Autodesk Inventor part; units mm, degrees
(part 2 of 3)
  line L434 (6.5872, -21.6405) -> (5.7652, -19.2795)
  line L435 (1.8366, -22.5787) -> (2.09, -20.0135)
  line L436 (2.09, -20.0135) -> (2.4587, -19.9586)
  line L437 (2.4587, -19.9586) -> (3.2669, -21.9358)
  line L438 (3.2669, -21.9358) -> (3.4507, -19.8111)
  line L439 (3.4507, -19.8111) -> (3.8154, -19.7568)
  line L440 (3.8154, -19.7568) -> (4.8144, -22.1357)
  line L441 (4.8144, -22.1357) -> (4.4758, -22.1861)
  line L442 (4.4758, -22.1861) -> (3.6739, -20.21)
  line L443 (3.6739, -20.21) -> (3.4858, -22.3333)
  line L444 (3.4858, -22.3333) -> (3.1512, -22.3831)
  line L445 (3.1512, -22.3831) -> (2.3457, -20.383)
  line L446 (2.3457, -20.383) -> (2.1593, -22.5307)
  line L447 (2.1593, -22.5307) -> (1.8366, -22.5787)
  line L448 (1.4387, -20.0798) -> (0.6427, -22.5951)
  line L449 (0.6427, -22.5951) -> (0.2335, -22.6027)
  line L450 (0.2335, -22.6027) -> (-0.6558, -20.1189)
  line L451 (-0.6558, -20.1189) -> (-0.3054, -20.1124)
  line L452 (-0.3054, -20.1124) -> (-0.0655, -20.807)
  line L453 (-0.0655, -20.807) -> (0.8886, -20.7891)
  line L454 (0.8886, -20.7891) -> (1.1024, -20.0861)
  line L455 (1.1024, -20.0861) -> (1.4387, -20.0798)
  line L456 (0.031, -21.0888) -> (0.4398, -22.2585)
  line L457 (0.4398, -22.2585) -> (0.8027, -21.0744)
  line L458 (0.8027, -21.0744) -> (0.031, -21.0888)
  line L459 (-2.9434, -22.4342) -> (-1.873, -20.0164)
  line L460 (-1.873, -20.0164) -> (-1.5158, -20.0469)
  line L461 (-1.5158, -20.0469) -> (-0.8703, -22.611)
  line L462 (-0.8703, -22.611) -> (-1.2256, -22.5807)
  line L463 (-1.2256, -22.5807) -> (-1.7395, -20.4528)
  line L464 (-1.7395, -20.4528) -> (-2.6063, -22.4629)
  line L465 (-2.6063, -22.4629) -> (-2.9434, -22.4342)
  line L466 (-2.9935, -19.8918) -> (-3.4527, -22.3492)
  line L467 (-3.4527, -22.3492) -> (-4.9901, -22.0619)
  line L468 (-4.9901, -22.0619) -> (-4.9358, -21.7712)
  line L469 (-4.9358, -21.7712) -> (-3.725, -21.9974)
  line L470 (-3.725, -21.9974) -> (-3.5992, -21.3243)
  line L471 (-3.5992, -21.3243) -> (-4.7284, -21.1133)
  line L472 (-4.7284, -21.1133) -> (-4.674, -20.8226)
  line L473 (-4.674, -20.8226) -> (-3.5449, -21.0336)
  line L474 (-3.5449, -21.0336) -> (-3.3744, -20.1215)
  line L475 (-3.3744, -20.1215) -> (-4.5852, -19.8952)
  line L476 (-4.5852, -19.8952) -> (-4.5309, -19.6045)
  line L477 (-4.5309, -19.6045) -> (-2.9935, -19.8918)
  line L478 (-7.744, -18.5856) -> (-7.337, -18.7292)
  line L479 (-7.337, -18.7292) -> (-6.9228, -19.93)
  line L480 (-6.9228, -19.93) -> (-6.5636, -20.0567)
  line L481 (-6.5636, -20.0567) -> (-6.2327, -19.1186)
  line L482 (-6.2327, -19.1186) -> (-5.9194, -19.2291)
  line L483 (-5.9194, -19.2291) -> (-6.7509, -21.5868)
  line L484 (-6.7509, -21.5868) -> (-7.3585, -21.3725)
  spline S195 degree 2 poles (-7.3585, -21.3725) (-7.561, -21.3011) (-7.8187, -21.1608) (-7.9146, -21.0367) knots 0 0 0 1 2 2 2
  spline S196 degree 2 poles (-7.9146, -21.0367) (-8.0105, -20.9127) (-8.0655, -20.6119) (-8.0001, -20.4266) knots 0 0 0 1 2 2 2
  spline S197 degree 2 poles (-8.0001, -20.4266) (-7.9092, -20.1686) (-7.5222, -19.912) (-7.2671, -19.9074) knots 0 0 0 1 2 2 2
  line L485 (-7.2671, -19.9074) -> (-7.744, -18.5856)
  spline S198 degree 2 poles (-7.6647, -20.5169) (-7.7011, -20.6201) (-7.6844, -20.8043) (-7.6261, -20.8828) knots 0 0 0 1 2 2 2
  spline S199 degree 2 poles (-7.6261, -20.8828) (-7.5748, -20.9504) (-7.4099, -21.0493) (-7.28, -21.0952) knots 0 0 0 1 2 2 2
  line L486 (-7.28, -21.0952) -> (-6.9685, -21.205)
  line L487 (-6.9685, -21.205) -> (-6.6559, -20.3185)
  line L488 (-6.6559, -20.3185) -> (-6.931, -20.2214)
  spline S200 degree 2 poles (-6.931, -20.2214) (-7.0667, -20.1736) (-7.2994, -20.1452) (-7.4002, -20.1935) knots 0 0 0 1 2 2 2
  spline S201 degree 2 poles (-7.4002, -20.1935) (-7.4919, -20.2342) (-7.6215, -20.3947) (-7.6647, -20.5169) knots 0 0 0 1 2 2 2
  line L489 (-7.9195, -18.4912) -> (-8.9844, -20.753)
  line L490 (-8.9844, -20.753) -> (-10.3995, -20.0869)
  line L491 (-10.3995, -20.0869) -> (-10.2735, -19.8192)
  line L492 (-10.2735, -19.8192) -> (-9.159, -20.3439)
  line L493 (-9.159, -20.3439) -> (-8.8674, -19.7244)
  line L494 (-8.8674, -19.7244) -> (-9.9066, -19.2351)
  line L495 (-9.9066, -19.2351) -> (-9.7807, -18.9675)
  line L496 (-9.7807, -18.9675) -> (-8.7414, -19.4568)
  line L497 (-8.7414, -19.4568) -> (-8.3461, -18.6173)
  line L498 (-8.3461, -18.6173) -> (-9.4606, -18.0926)
  line L499 (-9.4606, -18.0926) -> (-9.3346, -17.825)
  line L500 (-9.3346, -17.825) -> (-7.9195, -18.4912)
  spline S202 degree 2 poles (-11.9895, -17.6987) (-11.8118, -17.4061) (-11.2884, -17.0792) (-11.0094, -17.0685) knots 0 0 0 1 2 2 2
  spline S203 degree 2 poles (-11.0094, -17.0685) (-10.7846, -17.0653) (-10.4083, -17.199) (-10.1486, -17.3568) knots 0 0 0 1 2 2 2
  line L501 (-10.1486, -17.3568) -> (-9.6568, -17.6555)
  line L502 (-9.6568, -17.6555) -> (-10.9548, -19.7922)
  line L503 (-10.9548, -19.7922) -> (-11.4413, -19.4966)
  spline S204 degree 2 poles (-11.4413, -19.4966) (-11.7426, -19.3136) (-12.0307, -19.0153) (-12.1036, -18.862) knots 0 0 0 1 2 2 2
  spline S205 degree 2 poles (-12.1036, -18.862) (-12.2265, -18.6001) (-12.1788, -18.0104) (-11.9895, -17.6987) knots 0 0 0 1 2 2 2
  spline S206 degree 2 poles (-11.6955, -17.882) (-11.8449, -18.1279) (-11.8935, -18.5748) (-11.7924, -18.7713) knots 0 0 0 1 2 2 2
  spline S207 degree 2 poles (-11.7924, -18.7713) (-11.7192, -18.9082) (-11.498, -19.1256) (-11.3058, -19.2423) knots 0 0 0 1 2 2 2
  line L504 (-11.3058, -19.2423) -> (-11.0894, -19.3738)
  line L505 (-11.0894, -19.3738) -> (-10.0902, -17.7289)
  line L506 (-10.0902, -17.7289) -> (-10.3066, -17.5974)
  spline S208 degree 2 poles (-10.3066, -17.5974) (-10.4953, -17.4827) (-10.8178, -17.3698) (-10.9833, -17.3807) knots 0 0 0 1 2 2 2
  spline S209 degree 2 poles (-10.9833, -17.3807) (-11.1932, -17.3907) (-11.5441, -17.6327) (-11.6955, -17.882) knots 0 0 0 1 2 2 2
  spline S210 degree 2 poles (-12.2898, -15.8424) (-12.1153, -15.9778) (-11.9268, -16.2702) (-11.9064, -16.4322) knots 0 0 0 1 2 2 2
  spline S211 degree 2 poles (-11.9064, -16.4322) (-11.8818, -16.6154) (-12.0205, -16.9693) (-12.1844, -17.1806) knots 0 0 0 1 2 2 2
  line L507 (-12.1844, -17.1806) -> (-13.1407, -18.4132)
  line L508 (-13.1407, -18.4132) -> (-13.4032, -18.2095)
  line L509 (-13.4032, -18.2095) -> (-12.4469, -16.977)
  spline S212 degree 2 poles (-12.4469, -16.977) (-12.3401, -16.8393) (-12.2313, -16.6263) (-12.2225, -16.5126) knots 0 0 0 1 2 2 2
  spline S213 degree 2 poles (-12.2225, -16.5126) (-12.2133, -16.3916) (-12.3324, -16.1684) (-12.4637, -16.0665) knots 0 0 0 1 2 2 2
  spline S214 degree 2 poles (-12.4637, -16.0665) (-12.5869, -15.9709) (-12.8423, -15.9035) (-12.9573, -15.9426) knots 0 0 0 1 2 2 2
  spline S215 degree 2 poles (-12.9573, -15.9426) (-13.0652, -15.9793) (-13.2433, -16.1361) (-13.3464, -16.2689) knots 0 0 0 1 2 2 2
  line L510 (-13.3464, -16.2689) -> (-14.3076, -17.5078)
  line L511 (-14.3076, -17.5078) -> (-14.5701, -17.3042)
  line L512 (-14.5701, -17.3042) -> (-13.6138, -16.0717)
  spline S216 degree 2 poles (-13.6138, -16.0717) (-13.4536, -15.8652) (-13.1419, -15.6352) (-12.958, -15.6163) knots 0 0 0 1 2 2 2
  spline S217 degree 2 poles (-12.958, -15.6163) (-12.7915, -15.5968) (-12.4723, -15.7009) (-12.2898, -15.8424) knots 0 0 0 1 2 2 2
  spline S218 degree 2 poles (-14.0647, -14.3028) (-13.8897, -14.4716) (-13.7075, -14.8752) (-13.7135, -15.0974) knots 0 0 0 1 2 2 2
  spline S219 degree 2 poles (-13.7135, -15.0974) (-13.718, -15.3181) (-13.9374, -15.782) (-14.1568, -16.0095) knots 0 0 0 1 2 2 2
  spline S220 degree 2 poles (-14.1568, -16.0095) (-14.3747, -16.2356) (-14.8133, -16.46) (-15.0423, -16.4785) knots 0 0 0 1 2 2 2
  spline S221 degree 2 poles (-15.0423, -16.4785) (-15.2669, -16.4955) (-15.6838, -16.3383) (-15.8661, -16.1625) knots 0 0 0 1 2 2 2
  spline S222 degree 2 poles (-15.8661, -16.1625) (-15.9566, -16.0753) (-16.0902, -15.8958) (-16.1376, -15.8107) knots 0 0 0 1 2 2 2
  spline S223 degree 2 poles (-16.1376, -15.8107) (-16.1777, -15.7355) (-16.2467, -15.5648) (-16.2756, -15.4751) knots 0 0 0 1 2 2 2
  line L513 (-16.2756, -15.4751) -> (-15.9971, -15.1863)
  line L514 (-15.9971, -15.1863) -> (-15.9782, -15.2046)
  spline S224 degree 2 poles (-15.9782, -15.2046) (-15.9742, -15.2647) (-15.9538, -15.442) (-15.9203, -15.5503) knots 0 0 0 1 2 2 2
  spline S225 degree 2 poles (-15.9203, -15.5503) (-15.8883, -15.6543) (-15.7728, -15.8585) (-15.6678, -15.9597) knots 0 0 0 1 2 2 2
  spline S226 degree 2 poles (-15.6678, -15.9597) (-15.5526, -16.0708) (-15.2556, -16.1743) (-15.0911, -16.1584) knots 0 0 0 1 2 2 2
  spline S227 degree 2 poles (-15.0911, -16.1584) (-14.9267, -16.1396) (-14.5735, -15.9426) (-14.4061, -15.7691) knots 0 0 0 1 2 2 2
  spline S228 degree 2 poles (-14.4061, -15.7691) (-14.2276, -15.5839) (-14.0592, -15.2312) (-14.0479, -15.0648) knots 0 0 0 1 2 2 2
  spline S229 degree 2 poles (-14.0479, -15.0648) (-14.038, -14.9027) (-14.1535, -14.6168) (-14.2673, -14.5071) knots 0 0 0 1 2 2 2
  spline S230 degree 2 poles (-14.2673, -14.5071) (-14.3708, -14.4073) (-14.5965, -14.2882) (-14.7016, -14.26) knots 0 0 0 1 2 2 2
  spline S231 degree 2 poles (-14.7016, -14.26) (-14.8038, -14.2347) (-14.9775, -14.2192) (-15.0319, -14.2202) knots 0 0 0 1 2 2 2
  line L515 (-15.0319, -14.2202) -> (-15.0494, -14.2033)
  line L516 (-15.0494, -14.2033) -> (-14.7738, -13.9175)
  spline S232 degree 2 poles (-14.7738, -13.9175) (-14.6873, -13.9474) (-14.533, -13.9976) (-14.4362, -14.046) knots 0 0 0 1 2 2 2
  spline S233 degree 2 poles (-14.4362, -14.046) (-14.3321, -14.0957) (-14.1726, -14.1988) (-14.0647, -14.3028) knots 0 0 0 1 2 2 2
  line L517 (-14.858, -13.5603) -> (-16.763, -15.1793)
  line L518 (-16.763, -15.1793) -> (-17.7758, -13.9875)
  line L519 (-17.7758, -13.9875) -> (-17.5505, -13.7959)
  line L520 (-17.5505, -13.7959) -> (-16.7528, -14.7345)
  line L521 (-16.7528, -14.7345) -> (-16.231, -14.2911)
  line L522 (-16.231, -14.2911) -> (-16.9749, -13.4158)
  line L523 (-16.9749, -13.4158) -> (-16.7495, -13.2243)
  line L524 (-16.7495, -13.2243) -> (-16.0056, -14.0996)
  line L525 (-16.0056, -14.0996) -> (-15.2986, -13.4987)
  line L526 (-15.2986, -13.4987) -> (-16.0962, -12.5601)
  line L527 (-16.0962, -12.5601) -> (-15.8709, -12.3685)
  line L528 (-15.8709, -12.3685) -> (-14.858, -13.5603)
  line L529 (-17.1888, -10.4852) -> (-16.9439, -10.8405)
  line L530 (-16.9439, -10.8405) -> (-17.3146, -12.0556)
  line L531 (-17.3146, -12.0556) -> (-17.0984, -12.3692)
  line L532 (-17.0984, -12.3692) -> (-16.2794, -11.8047)
  line L533 (-16.2794, -11.8047) -> (-16.0908, -12.0783)
  line L534 (-16.0908, -12.0783) -> (-18.1493, -13.497)
  line L535 (-18.1493, -13.497) -> (-18.5149, -12.9666)
  spline S234 degree 2 poles (-18.5149, -12.9666) (-18.6367, -12.7897) (-18.7628, -12.5248) (-18.7674, -12.368) knots 0 0 0 1 2 2 2
  spline S235 degree 2 poles (-18.7674, -12.368) (-18.7721, -12.2113) (-18.6398, -11.9356) (-18.478, -11.8241) knots 0 0 0 1 2 2 2
  spline S236 degree 2 poles (-18.478, -11.8241) (-18.2528, -11.6689) (-17.7889, -11.6887) (-17.5798, -11.8349) knots 0 0 0 1 2 2 2
  line L536 (-17.5798, -11.8349) -> (-17.1888, -10.4852)
  spline S237 degree 2 poles (-18.2597, -12.0944) (-18.3498, -12.1565) (-18.4446, -12.3153) (-18.4436, -12.4131) knots 0 0 0 1 2 2 2
  spline S238 degree 2 poles (-18.4436, -12.4131) (-18.4417, -12.4979) (-18.3665, -12.6749) (-18.2883, -12.7883) knots 0 0 0 1 2 2 2
  line L537 (-18.2883, -12.7883) -> (-18.1009, -13.0602)
  line L538 (-18.1009, -13.0602) -> (-17.3269, -12.5267)
  line L539 (-17.3269, -12.5267) -> (-17.4925, -12.2865)
  spline S239 degree 2 poles (-17.4925, -12.2865) (-17.5741, -12.1681) (-17.7457, -12.0083) (-17.8556, -11.9881) knots 0 0 0 1 2 2 2
  spline S240 degree 2 poles (-17.8556, -11.9881) (-17.9537, -11.9671) (-18.153, -12.0208) (-18.2597, -12.0944) knots 0 0 0 1 2 2 2
  line L540 (-20.4598, -8.1233) -> (-18.5574, -7.7669)
  line L541 (-18.5574, -7.7669) -> (-18.4348, -8.0316)
  line L542 (-18.4348, -8.0316) -> (-19.5549, -9.055)
  line L543 (-19.5549, -9.055) -> (-18.0508, -8.8607)
  line L544 (-18.0508, -8.8607) -> (-17.9291, -9.1236)
  line L545 (-17.9291, -9.1236) -> (-19.4296, -10.3477)
  line L546 (-19.4296, -10.3477) -> (-19.5675, -10.0499)
  line L547 (-19.5675, -10.0499) -> (-18.389, -9.1379)
  line L548 (-18.389, -9.1379) -> (-19.8936, -9.3458)
  line L549 (-19.8936, -9.3458) -> (-20.0034, -9.1086)
  line L550 (-20.0034, -9.1086) -> (-18.8769, -8.0846)
  line L551 (-18.8769, -8.0846) -> (-20.3261, -8.4119)
  line L552 (-20.3261, -8.4119) -> (-20.4598, -8.1233)
  line L553 (-18.9331, -6.76) -> (-18.8245, -7.0568)
  line L554 (-18.8245, -7.0568) -> (-20.5863, -7.7015)
  line L555 (-20.5863, -7.7015) -> (-20.6949, -7.4047)
  line L556 (-20.6949, -7.4047) -> (-18.9331, -6.76)
  line L557 (-20.9956, -7.491) -> (-20.8723, -7.8278)
  line L558 (-20.8723, -7.8278) -> (-21.1805, -7.9406)
  line L559 (-21.1805, -7.9406) -> (-21.3038, -7.6038)
  line L560 (-21.3038, -7.6038) -> (-20.9956, -7.491)
  spline S241 degree 2 poles (-19.2205, -5.7699) (-19.1439, -6.0155) (-19.3379, -6.3796) (-19.6415, -6.4744) knots 0 0 0 1 2 2 2
  line L561 (-19.6415, -6.4744) -> (-20.6336, -6.7842)
  line L562 (-20.6336, -6.7842) -> (-20.5702, -6.9872)
  line L563 (-20.5702, -6.9872) -> (-20.8197, -7.0651)
  line L564 (-20.8197, -7.0651) -> (-20.8831, -6.862)
  line L565 (-20.8831, -6.862) -> (-21.3975, -7.0227)
  line L566 (-21.3975, -7.0227) -> (-21.4917, -6.721)
  line L567 (-21.4917, -6.721) -> (-20.9773, -6.5604)
  line L568 (-20.9773, -6.5604) -> (-21.1506, -6.0053)
  line L569 (-21.1506, -6.0053) -> (-20.9011, -5.9275)
  line L570 (-20.9011, -5.9275) -> (-20.7278, -6.4825)
  line L571 (-20.7278, -6.4825) -> (-19.875, -6.2162)
  spline S242 degree 2 poles (-19.875, -6.2162) (-19.7396, -6.1739) (-19.5937, -6.1178) (-19.5402, -6.065) knots 0 0 0 1 2 2 2
  spline S243 degree 2 poles (-19.5402, -6.065) (-19.4925, -6.0204) (-19.4745, -5.881) (-19.5071, -5.7766) knots 0 0 0 1 2 2 2
  spline S244 degree 2 poles (-19.5071, -5.7766) (-19.53, -5.7031) (-19.6174, -5.5797) (-19.6406, -5.553) knots 0 0 0 1 2 2 2
  line L572 (-19.6406, -5.553) -> (-19.646, -5.5356)
  line L573 (-19.646, -5.5356) -> (-19.3753, -5.451)
  spline S245 degree 2 poles (-19.3753, -5.451) (-19.3255, -5.5289) (-19.2441, -5.6945) (-19.2205, -5.7699) knots 0 0 0 1 2 2 2
  line L574 (-19.7571, -3.7879) -> (-19.6861, -4.0959)
  line L575 (-19.6861, -4.0959) -> (-20.7285, -4.336)
  spline S246 degree 2 poles (-20.7285, -4.336) (-20.8549, -4.3651) (-21.0666, -4.4389) (-21.1235, -4.4894) knots 0 0 0 1 2 2 2
  spline S247 degree 2 poles (-21.1235, -4.4894) (-21.184, -4.5428) (-21.2202, -4.6925) (-21.1938, -4.807) knots 0 0 0 1 2 2 2
  spline S248 degree 2 poles (-21.1938, -4.807) (-21.1674, -4.9215) (-20.9891, -5.1362) (-20.8636, -5.2299) knots 0 0 0 1 2 2 2
  line L576 (-20.8636, -5.2299) -> (-19.4974, -4.9152)
  line L577 (-19.4974, -4.9152) -> (-19.4265, -5.2232)
  line L578 (-19.4265, -5.2232) -> (-21.9712, -5.8094)
  line L579 (-21.9712, -5.8094) -> (-22.0422, -5.5014)
  line L580 (-22.0422, -5.5014) -> (-21.1222, -5.2895)
  spline S249 degree 2 poles (-21.1222, -5.2895) (-21.2784, -5.1799) (-21.4701, -4.9434) (-21.5047, -4.7934) knots 0 0 0 1 2 2 2
  spline S250 degree 2 poles (-21.5047, -4.7934) (-21.5665, -4.5249) (-21.2812, -4.139) (-20.9436, -4.0612) knots 0 0 0 1 2 2 2
  line L581 (-20.9436, -4.0612) -> (-19.7571, -3.7879)
  spline S251 degree 2 poles (-20.0182, -1.2873) (-20.0002, -1.5297) (-20.1335, -1.952) (-20.286, -2.1137) knots 0 0 0 1 2 2 2
  spline S252 degree 2 poles (-20.286, -2.1137) (-20.4365, -2.2752) (-20.9093, -2.4748) (-21.2245, -2.4982) knots 0 0 0 1 2 2 2
  spline S253 degree 2 poles (-21.2245, -2.4982) (-21.5376, -2.5214) (-22.0142, -2.3963) (-22.1971, -2.2575) knots 0 0 0 1 2 2 2
  spline S254 degree 2 poles (-22.1971, -2.2575) (-22.3759, -2.1204) (-22.582, -1.7254) (-22.6007, -1.4728) knots 0 0 0 1 2 2 2
  spline S255 degree 2 poles (-22.6007, -1.4728) (-22.61, -1.3475) (-22.59, -1.1246) (-22.5686, -1.0296) knots 0 0 0 1 2 2 2
  spline S256 degree 2 poles (-22.5686, -1.0296) (-22.5483, -0.9468) (-22.486, -0.7736) (-22.4477, -0.6875) knots 0 0 0 1 2 2 2
  line L582 (-22.4477, -0.6875) -> (-22.0477, -0.6578)
  line L583 (-22.0477, -0.6578) -> (-22.0457, -0.684)
  spline S257 degree 2 poles (-22.0457, -0.684) (-22.0828, -0.7315) (-22.1858, -0.8773) (-22.233, -0.9803) knots 0 0 0 1 2 2 2
  spline S258 degree 2 poles (-22.233, -0.9803) (-22.2785, -1.0792) (-22.3285, -1.3084) (-22.3177, -1.4538) knots 0 0 0 1 2 2 2
  spline S259 degree 2 poles (-22.3177, -1.4538) (-22.3059, -1.6135) (-22.1534, -1.8886) (-22.0202, -1.9864) knots 0 0 0 1 2 2 2
  spline S260 degree 2 poles (-22.0202, -1.9864) (-21.8851, -2.082) (-21.4905, -2.1705) (-21.2501, -2.1527) knots 0 0 0 1 2 2 2
  spline S261 degree 2 poles (-21.2501, -2.1527) (-20.9935, -2.1337) (-20.6329, -1.983) (-20.5136, -1.8665) knots 0 0 0 1 2 2 2
  spline S262 degree 2 poles (-20.5136, -1.8665) (-20.3981, -1.7522) (-20.2937, -1.4621) (-20.3054, -1.3045) knots 0 0 0 1 2 2 2
  spline S263 degree 2 poles (-20.3054, -1.3045) (-20.3161, -1.1611) (-20.4049, -0.9219) (-20.4645, -0.8308) knots 0 0 0 1 2 2 2
  spline S264 degree 2 poles (-20.4645, -0.8308) (-20.5238, -0.7438) (-20.6429, -0.6165) (-20.6841, -0.581) knots 0 0 0 1 2 2 2
  line L584 (-20.6841, -0.581) -> (-20.6859, -0.5567)
  line L585 (-20.6859, -0.5567) -> (-20.2899, -0.5273)
  spline S265 degree 2 poles (-20.2899, -0.5273) (-20.2454, -0.6073) (-20.1639, -0.7476) (-20.1239, -0.8482) knots 0 0 0 1 2 2 2
  spline S266 degree 2 poles (-20.1239, -0.8482) (-20.0795, -0.9546) (-20.0293, -1.1378) (-20.0182, -1.2873) knots 0 0 0 1 2 2 2
  line L586 (-20.0601, 1.7288) -> (-20.0731, 1.2975)
  line L587 (-20.0731, 1.2975) -> (-21.0913, 0.5378)
  line L588 (-21.0913, 0.5378) -> (-21.1028, 0.1571)
  line L589 (-21.1028, 0.1571) -> (-20.1085, 0.127)
  line L590 (-20.1085, 0.127) -> (-20.1186, -0.2051)
  line L591 (-20.1186, -0.2051) -> (-22.6174, -0.1295)
  line L592 (-22.6174, -0.1295) -> (-22.5979, 0.5145)
  spline S267 degree 2 poles (-22.5979, 0.5145) (-22.5914, 0.7291) (-22.5361, 1.0173) (-22.4471, 1.1463) knots 0 0 0 1 2 2 2
  spline S268 degree 2 poles (-22.4471, 1.1463) (-22.358, 1.2754) (-22.0882, 1.4192) (-21.8918, 1.4133) knots 0 0 0 1 2 2 2
  spline S269 degree 2 poles (-21.8918, 1.4133) (-21.6184, 1.405) (-21.2563, 1.1143) (-21.1744, 0.8727) knots 0 0 0 1 2 2 2
  line L593 (-21.1744, 0.8727) -> (-20.0601, 1.7288)
  spline S270 degree 2 poles (-21.8759, 1.0662) (-21.9853, 1.0695) (-22.1557, 0.9977) (-22.2128, 0.9183) knots 0 0 0 1 2 2 2
  spline S271 degree 2 poles (-22.2128, 0.9183) (-22.2615, 0.8488) (-22.3057, 0.6617) (-22.3098, 0.524) knots 0 0 0 1 2 2 2
  line L594 (-22.3098, 0.524) -> (-22.3198, 0.1939)
  line L595 (-22.3198, 0.1939) -> (-21.3802, 0.1655)
  line L596 (-21.3802, 0.1655) -> (-21.3714, 0.4571)
  spline S272 degree 2 poles (-21.3714, 0.4571) (-21.3671, 0.6009) (-21.4108, 0.8312) (-21.4873, 0.9126) knots 0 0 0 1 2 2 2
  spline S273 degree 2 poles (-21.4873, 0.9126) (-21.554, 0.9876) (-21.7463, 1.0623) (-21.8759, 1.0662) knots 0 0 0 1 2 2 2
  spline S274 degree 2 poles (-21.9722, 3.993) (-21.7874, 4.1095) (-21.2836, 4.1963) (-20.9748, 4.1516) knots 0 0 0 1 2 2 2
  spline S275 degree 2 poles (-20.9748, 4.1516) (-20.6741, 4.1081) (-20.2089, 3.8852) (-20.0654, 3.717) knots 0 0 0 1 2 2 2
  spline S276 degree 2 poles (-20.0654, 3.717) (-19.915, 3.5397) (-19.8089, 3.1129) (-19.844, 2.8703) knots 0 0 0 1 2 2 2
  spline S277 degree 2 poles (-19.844, 2.8703) (-19.8802, 2.6197) (-20.1087, 2.2433) (-20.2963, 2.121) knots 0 0 0 1 2 2 2
  spline S278 degree 2 poles (-20.2963, 2.121) (-20.4813, 2.0025) (-20.9866, 1.92) (-21.2913, 1.9641) knots 0 0 0 1 2 2 2
  spline S279 degree 2 poles (-21.2913, 1.9641) (-21.6021, 2.0091) (-22.053, 2.2319) (-22.2028, 2.3989) knots 0 0 0 1 2 2 2
  spline S280 degree 2 poles (-22.2028, 2.3989) (-22.3463, 2.5671) (-22.4585, 2.9948) (-22.4225, 3.2434) knots 0 0 0 1 2 2 2
  spline S281 degree 2 poles (-22.4225, 3.2434) (-22.3859, 3.496) (-22.1509, 3.8755) (-21.9722, 3.993) knots 0 0 0 1 2 2 2
  spline S282 degree 2 poles (-21.0244, 3.8087) (-21.2691, 3.8441) (-21.6634, 3.7927) (-21.8016, 3.7144) knots 0 0 0 1 2 2 2
  spline S283 degree 2 poles (-21.8016, 3.7144) (-21.9442, 3.6348) (-22.1125, 3.3766) (-22.1375, 3.2042) knots 0 0 0 1 2 2 2
  spline S284 degree 2 poles (-22.1375, 3.2042) (-22.1633, 3.0258) (-22.0779, 2.7391) (-21.9603, 2.6177) knots 0 0 0 1 2 2 2
  spline S285 degree 2 poles (-21.9603, 2.6177) (-21.8482, 2.5012) (-21.4823, 2.3418) (-21.2417, 2.307) knots 0 0 0 1 2 2 2
  spline S286 degree 2 poles (-21.2417, 2.307) (-20.7545, 2.2365) (-20.178, 2.5706) (-20.1284, 2.9135) knots 0 0 0 1 2 2 2
  spline S287 degree 2 poles (-20.1284, 2.9135) (-20.0788, 3.2564) (-20.5372, 3.7382) (-21.0244, 3.8087) knots 0 0 0 1 2 2 2
  spline S288 degree 2 poles (-19.4282, 4.9892) (-19.4958, 4.7262) (-19.7006, 4.3856) (-19.8209, 4.243) knots 0 0 0 1 2 2 2
  line L597 (-19.8209, 4.243) -> (-20.2251, 4.3469)
  line L598 (-20.2251, 4.3469) -> (-20.2191, 4.3704)
  spline S289 degree 2 poles (-20.2191, 4.3704) (-20.0291, 4.491) (-19.7608, 4.8509) (-19.7129, 5.0373) knots 0 0 0 1 2 2 2
  spline S290 degree 2 poles (-19.7129, 5.0373) (-19.6443, 5.3041) (-19.7958, 5.6339) (-19.9783, 5.6808) knots 0 0 0 1 2 2 2
  spline S291 degree 2 poles (-19.9783, 5.6808) (-20.1235, 5.7181) (-20.3409, 5.6213) (-20.4258, 5.4779) knots 0 0 0 1 2 2 2
  spline S292 degree 2 poles (-20.4258, 5.4779) (-20.486, 5.3742) (-20.5771, 5.1989) (-20.6482, 5.0686) knots 0 0 0 1 2 2 2
  spline S293 degree 2 poles (-20.6482, 5.0686) (-20.7139, 4.9516) (-20.8649, 4.7792) (-20.9651, 4.7234) knots 0 0 0 1 2 2 2
  spline S294 degree 2 poles (-20.9651, 4.7234) (-21.0647, 4.6695) (-21.3017, 4.6426) (-21.443, 4.6789) knots 0 0 0 1 2 2 2
  spline S295 degree 2 poles (-21.443, 4.6789) (-21.7373, 4.7546) (-22.0175, 5.3162) (-21.9262, 5.6713) knots 0 0 0 1 2 2 2
  spline S296 degree 2 poles (-21.9262, 5.6713) (-21.8737, 5.8754) (-21.7004, 6.2157) (-21.584, 6.351) knots 0 0 0 1 2 2 2
  line L599 (-21.584, 6.351) -> (-21.1995, 6.2521)
  line L600 (-21.1995, 6.2521) -> (-21.2055, 6.2286)
  spline S297 degree 2 poles (-21.2055, 6.2286) (-21.3412, 6.1401) (-21.591, 5.8194) (-21.642, 5.6212) knots 0 0 0 1 2 2 2
  spline S298 degree 2 poles (-21.642, 5.6212) (-21.6995, 5.3976) (-21.5607, 5.0669) (-21.39, 5.023) knots 0 0 0 1 2 2 2
  spline S299 degree 2 poles (-21.39, 5.023) (-21.237, 4.9837) (-21.0126, 5.0996) (-20.9321, 5.242) knots 0 0 0 1 2 2 2
  spline S300 degree 2 poles (-20.9321, 5.242) (-20.8784, 5.337) (-20.7315, 5.6151) (-20.6769, 5.7056) knots 0 0 0 1 2 2 2
  spline S301 degree 2 poles (-20.6769, 5.7056) (-20.5363, 5.9351) (-20.1687, 6.0875) (-19.943, 6.0294) knots 0 0 0 1 2 2 2
  spline S302 degree 2 poles (-19.943, 6.0294) (-19.7998, 5.9926) (-19.5549, 5.8062) (-19.4855, 5.6775) knots 0 0 0 1 2 2 2
  spline S303 degree 2 poles (-19.4855, 5.6775) (-19.4093, 5.5345) (-19.3712, 5.2109) (-19.4282, 4.9892) knots 0 0 0 1 2 2 2
  spline S304 degree 2 poles (-18.8663, 6.8126) (-18.9585, 6.5573) (-19.1947, 6.2377) (-19.3281, 6.1071) knots 0 0 0 1 2 2 2
  line L601 (-19.3281, 6.1071) -> (-19.7206, 6.249)
  line L602 (-19.7206, 6.249) -> (-19.7123, 6.2719)
  spline S305 degree 2 poles (-19.7123, 6.2719) (-19.5117, 6.3738) (-19.2105, 6.7066) (-19.1451, 6.8876) knots 0 0 0 1 2 2 2
  spline S306 degree 2 poles (-19.1451, 6.8876) (-19.0514, 7.1467) (-19.171, 7.4893) (-19.3481, 7.5534) knots 0 0 0 1 2 2 2
  spline S307 degree 2 poles (-19.3481, 7.5534) (-19.4891, 7.6044) (-19.7147, 7.5286) (-19.8129, 7.394) knots 0 0 0 1 2 2 2
  spline S308 degree 2 poles (-19.8129, 7.394) (-19.8827, 7.2964) (-19.99, 7.1305) (-20.0732, 7.0077) knots 0 0 0 1 2 2 2
  spline S309 degree 2 poles (-20.0732, 7.0077) (-20.1497, 6.8974) (-20.3164, 6.7401) (-20.4214, 6.6941) knots 0 0 0 1 2 2 2
  spline S310 degree 2 poles (-20.4214, 6.6941) (-20.5257, 6.6499) (-20.7642, 6.6456) (-20.9014, 6.6952) knots 0 0 0 1 2 2 2
  spline S311 degree 2 poles (-20.9014, 6.6952) (-21.1872, 6.7986) (-21.4128, 7.3842) (-21.2881, 7.7291) knots 0 0 0 1 2 2 2
  spline S312 degree 2 poles (-21.2881, 7.7291) (-21.2165, 7.9272) (-21.0116, 8.2495) (-20.8829, 8.3732) knots 0 0 0 1 2 2 2
  line L603 (-20.8829, 8.3732) -> (-20.5095, 8.2382)
  line L604 (-20.5095, 8.2382) -> (-20.5177, 8.2153)
  spline S313 degree 2 poles (-20.5177, 8.2153) (-20.6613, 8.1401) (-20.9404, 7.8446) (-21.01, 7.6522) knots 0 0 0 1 2 2 2
  spline S314 degree 2 poles (-21.01, 7.6522) (-21.0885, 7.435) (-20.9817, 7.0927) (-20.816, 7.0327) knots 0 0 0 1 2 2 2
  spline S315 degree 2 poles (-20.816, 7.0327) (-20.6674, 6.979) (-20.433, 7.0731) (-20.3393, 7.2073) knots 0 0 0 1 2 2 2
  spline S316 degree 2 poles (-20.3393, 7.2073) (-20.2768, 7.2967) (-20.1042, 7.5596) (-20.0412, 7.6445) knots 0 0 0 1 2 2 2
  spline S317 degree 2 poles (-20.0412, 7.6445) (-19.8794, 7.8596) (-19.499, 7.9763) (-19.2799, 7.8971) knots 0 0 0 1 2 2 2
  spline S318 degree 2 poles (-19.2799, 7.8971) (-19.1408, 7.8468) (-18.9147, 7.638) (-18.8579, 7.5033) knots 0 0 0 1 2 2 2
  spline S319 degree 2 poles (-18.8579, 7.5033) (-18.7956, 7.3537) (-18.7884, 7.0279) (-18.8663, 6.8126) knots 0 0 0 1 2 2 2
  line L605 (-17.0953, 10.637) -> (-17.3025, 10.2585)
  line L606 (-17.3025, 10.2585) -> (-18.5545, 10.0431)
  line L607 (-18.5545, 10.0431) -> (-18.7374, 9.709)
  line L608 (-18.7374, 9.709) -> (-17.8648, 9.2313)
  line L609 (-17.8648, 9.2313) -> (-18.0244, 8.9399)
  line L610 (-18.0244, 8.9399) -> (-20.2173, 10.1403)
  line L611 (-20.2173, 10.1403) -> (-19.9079, 10.7055)
  spline S320 degree 2 poles (-19.9079, 10.7055) (-19.8048, 10.8938) (-19.6248, 11.1256) (-19.4869, 11.2002) knots 0 0 0 1 2 2 2
  spline S321 degree 2 poles (-19.4869, 11.2002) (-19.3491, 11.2749) (-19.0433, 11.2807) (-18.8709, 11.1864) knots 0 0 0 1 2 2 2
  spline S322 degree 2 poles (-18.8709, 11.1864) (-18.631, 11.055) (-18.4401, 10.6318) (-18.4767, 10.3793) knots 0 0 0 1 2 2 2
  line L612 (-18.4767, 10.3793) -> (-17.0953, 10.637)
  spline S323 degree 2 poles (-19.0142, 10.8698) (-19.1101, 10.9224) (-19.2946, 10.9356) (-19.3815, 10.8908) knots 0 0 0 1 2 2 2
  spline S324 degree 2 poles (-19.3815, 10.8908) (-19.4564, 10.8509) (-19.5807, 10.7042) (-19.6468, 10.5833) knots 0 0 0 1 2 2 2
  line L613 (-19.6468, 10.5833) -> (-19.8054, 10.2936)
  line L614 (-19.8054, 10.2936) -> (-18.9808, 9.8423)
  line L615 (-18.9808, 9.8423) -> (-18.8407, 10.0982)
  spline S325 degree 2 poles (-18.8407, 10.0982) (-18.7717, 10.2243) (-18.7062, 10.4495) (-18.7375, 10.5567) knots 0 0 0 1 2 2 2
  spline S326 degree 2 poles (-18.7375, 10.5567) (-18.7629, 10.6538) (-18.9004, 10.8076) (-19.0142, 10.8698) knots 0 0 0 1 2 2 2
  spline S327 degree 2 poles (-17.7729, 13.522) (-17.5554, 13.5422) (-17.0669, 13.391) (-16.812, 13.2112) knots 0 0 0 1 2 2 2
  spline S328 degree 2 poles (-16.812, 13.2112) (-16.5637, 13.036) (-16.2501, 12.6264) (-16.1985, 12.4115) knots 0 0 0 1 2 2 2
  spline S329 degree 2 poles (-16.1985, 12.4115) (-16.1448, 12.1852) (-16.2438, 11.7567) (-16.3851, 11.5564) knots 0 0 0 1 2 2 2
  spline S330 degree 2 poles (-16.3851, 11.5564) (-16.5311, 11.3495) (-16.9053, 11.1176) (-17.128, 11.0937) knots 0 0 0 1 2 2 2
  spline S331 degree 2 poles (-17.128, 11.0937) (-17.3467, 11.0719) (-17.8344, 11.2275) (-18.086, 11.405) knots 0 0 0 1 2 2 2
  spline S332 degree 2 poles (-18.086, 11.405) (-18.3426, 11.586) (-18.6434, 11.9891) (-18.7012, 12.2059) knots 0 0 0 1 2 2 2
  spline S333 degree 2 poles (-18.7012, 12.2059) (-18.7529, 12.4209) (-18.6589, 12.8529) (-18.5141, 13.0582) knots 0 0 0 1 2 2 2
  spline S334 degree 2 poles (-18.5141, 13.0582) (-18.367, 13.2668) (-17.9854, 13.4984) (-17.7729, 13.522) knots 0 0 0 1 2 2 2
  spline S335 degree 2 poles (-17.0117, 12.9281) (-17.2137, 13.0706) (-17.5884, 13.2035) (-17.7471, 13.1965) knots 0 0 0 1 2 2 2
  spline S336 degree 2 poles (-17.7471, 13.1965) (-17.9103, 13.1901) (-18.1774, 13.0364) (-18.2778, 12.894) knots 0 0 0 1 2 2 2
  spline S337 degree 2 poles (-18.2778, 12.894) (-18.3818, 12.7466) (-18.4356, 12.4524) (-18.3859, 12.2909) knots 0 0 0 1 2 2 2
  spline S338 degree 2 poles (-18.3859, 12.2909) (-18.3388, 12.1362) (-18.085, 11.8283) (-17.8863, 11.6881) knots 0 0 0 1 2 2 2
  spline S339 degree 2 poles (-17.8863, 11.6881) (-17.484, 11.4044) (-16.8187, 11.4408) (-16.619, 11.7239) knots 0 0 0 1 2 2 2
  spline S340 degree 2 poles (-16.619, 11.7239) (-16.4193, 12.007) (-16.6094, 12.6443) (-17.0117, 12.9281) knots 0 0 0 1 2 2 2
  line L616 (-14.5932, 13.8526) -> (-15.5453, 12.761)
  line L617 (-15.5453, 12.761) -> (-17.4293, 14.4043)
  line L618 (-17.4293, 14.4043) -> (-17.2109, 14.6547)
  line L619 (-17.2109, 14.6547) -> (-15.5498, 13.2058)
  line L620 (-15.5498, 13.2058) -> (-14.8161, 14.047)
  line L621 (-14.8161, 14.047) -> (-14.5932, 13.8526)
  line L622 (-13.3644, 15.0416) -> (-14.4058, 14.0347)
  line L623 (-14.4058, 14.0347) -> (-16.1435, 15.8321)
  line L624 (-16.1435, 15.8321) -> (-15.9046, 16.063)
  line L625 (-15.9046, 16.063) -> (-14.3725, 14.4783)
  line L626 (-14.3725, 14.4783) -> (-13.5699, 15.2542)
  line L627 (-13.5699, 15.2542) -> (-13.3644, 15.0416)
  line L628 (-13.1646, 15.2097) -> (-14.7329, 17.1567)
  line L629 (-14.7329, 17.1567) -> (-13.5148, 18.1378)
  line L630 (-13.5148, 18.1378) -> (-13.3293, 17.9074)
  line L631 (-13.3293, 17.9074) -> (-14.2886, 17.1348)
  line L632 (-14.2886, 17.1348) -> (-13.859, 16.6015)
  line L633 (-13.859, 16.6015) -> (-12.9644, 17.3221)
  line L634 (-12.9644, 17.3221) -> (-12.7789, 17.0917)
  line L635 (-12.7789, 17.0917) -> (-13.6735, 16.3711)
  line L636 (-13.6735, 16.3711) -> (-13.0914, 15.6485)
  line L637 (-13.0914, 15.6485) -> (-12.1321, 16.4212)
  line L638 (-12.1321, 16.4212) -> (-11.9466, 16.1909)
  line L639 (-11.9466, 16.1909) -> (-13.1646, 15.2097)
  line L640 (-10.0292, 17.4588) -> (-10.3909, 17.2233)
  line L641 (-10.3909, 17.2233) -> (-11.5958, 17.6258)
  line L642 (-11.5958, 17.6258) -> (-11.9149, 17.418)
  line L643 (-11.9149, 17.418) -> (-11.3722, 16.5844)
  line L644 (-11.3722, 16.5844) -> (-11.6506, 16.4031)
  line L645 (-11.6506, 16.4031) -> (-13.0147, 18.4982)
  line L646 (-13.0147, 18.4982) -> (-12.4748, 18.8497)
  spline S341 degree 2 poles (-12.4748, 18.8497) (-12.2948, 18.9669) (-12.0266, 19.0859) (-11.8699, 19.0864) knots 0 0 0 1 2 2 2
  spline S342 degree 2 poles (-11.8699, 19.0864) (-11.7131, 19.087) (-11.4409, 18.9475) (-11.3337, 18.7828) knots 0 0 0 1 2 2 2
  spline S343 degree 2 poles (-11.3337, 18.7828) (-11.1845, 18.5536) (-11.2165, 18.0904) (-11.3682, 17.8852) knots 0 0 0 1 2 2 2
  line L647 (-11.3682, 17.8852) -> (-10.0292, 17.4588)
  spline S344 degree 2 poles (-11.6097, 18.5717) (-11.6693, 18.6634) (-11.8256, 18.7623) (-11.9234, 18.7639) knots 0 0 0 1 2 2 2
  spline S345 degree 2 poles (-11.9234, 18.7639) (-12.0082, 18.7643) (-12.1871, 18.6937) (-12.3026, 18.6186) knots 0 0 0 1 2 2 2
  line L648 (-12.3026, 18.6186) -> (-12.5793, 18.4384)
  line L649 (-12.5793, 18.4384) -> (-12.0664, 17.6506)
  line L650 (-12.0664, 17.6506) -> (-11.8219, 17.8098)
  spline S346 degree 2 poles (-11.8219, 17.8098) (-11.7014, 17.8883) (-11.5371, 18.0556) (-11.514, 18.1649) knots 0 0 0 1 2 2 2
  spline S347 degree 2 poles (-11.514, 18.1649) (-11.4905, 18.2625) (-11.5389, 18.463) (-11.6097, 18.5717) knots 0 0 0 1 2 2 2
  spline S348 degree 2 poles (-7.6633, 19.4357) (-7.5873, 19.2656) (-7.6001, 18.9469) (-7.6694, 18.8139) knots 0 0 0 1 2 2 2
  spline S349 degree 2 poles (-7.6694, 18.8139) (-7.7542, 18.6561) (-8.0102, 18.4396) (-8.2433, 18.3354) knots 0 0 0 1 2 2 2
  line L651 (-8.2433, 18.3354) -> (-8.898, 18.0427)
  line L652 (-8.898, 18.0427) -> (-9.9183, 20.325)
  line L653 (-9.9183, 20.325) -> (-9.3135, 20.5954)
  spline S350 degree 2 poles (-9.3135, 20.5954) (-9.0694, 20.7046) (-8.8112, 20.7822) (-8.6729, 20.7708) knots 0 0 0 1 2 2 2
  spline S351 degree 2 poles (-8.6729, 20.7708) (-8.5201, 20.7615) (-8.3122, 20.5992) (-8.2477, 20.455) knots 0 0 0 1 2 2 2
  spline S352 degree 2 poles (-8.2477, 20.455) (-8.1757, 20.2941) (-8.2318, 19.9627) (-8.3494, 19.8236) knots 0 0 0 1 2 2 2
  line L654 (-8.3494, 19.8236) -> (-8.3444, 19.8125)
  spline S353 degree 2 poles (-8.3444, 19.8125) (-8.1162, 19.848) (-7.7609, 19.654) (-7.6633, 19.4357) knots 0 0 0 1 2 2 2
  spline S354 degree 2 poles (-7.9738, 19.2814) (-8.0317, 19.4109) (-8.1801, 19.5443) (-8.3175, 19.5538) knots 0 0 0 1 2 2 2
  spline S355 degree 2 poles (-8.3175, 19.5538) (-8.4062, 19.5586) (-8.5863, 19.5047) (-8.7435, 19.4344) knots 0 0 0 1 2 2 2
  line L655 (-8.7435, 19.4344) -> (-9.0875, 19.2806)
  line L656 (-9.0875, 19.2806) -> (-8.7105, 18.4372)
  line L657 (-8.7105, 18.4372) -> (-8.4645, 18.5472)
  spline S356 degree 2 poles (-8.4645, 18.5472) (-8.2647, 18.6365) (-8.0519, 18.776) (-7.9896, 18.8749) knots 0 0 0 1 2 2 2
  spline S357 degree 2 poles (-7.9896, 18.8749) (-7.9318, 18.974) (-7.9201, 19.1612) (-7.9738, 19.2814) knots 0 0 0 1 2 2 2
  spline S358 degree 2 poles (-8.5449, 20.271) (-8.5813, 20.3524) (-8.6914, 20.4497) (-8.7681, 20.4575) knots 0 0 0 1 2 2 2
  spline S359 degree 2 poles (-8.7681, 20.4575) (-8.8603, 20.4652) (-9.048, 20.4034) (-9.2089, 20.3315) knots 0 0 0 1 2 2 2
  line L658 (-9.2089, 20.3315) -> (-9.4992, 20.2017)
  line L659 (-9.4992, 20.2017) -> (-9.2008, 19.534)
  line L660 (-9.2008, 19.534) -> (-8.8567, 19.6878)
  spline S360 degree 2 poles (-8.8567, 19.6878) (-8.7143, 19.7515) (-8.5925, 19.8414) (-8.5411, 19.9199) knots 0 0 0 1 2 2 2
  spline S361 degree 2 poles (-8.5411, 19.9199) (-8.4906, 19.9957) (-8.497, 20.1638) (-8.5449, 20.271) knots 0 0 0 1 2 2 2
  line L661 (-7.0386, 18.8441) -> (-7.83, 21.2155)
  line L662 (-7.83, 21.2155) -> (-6.3464, 21.7107)
  line L663 (-6.3464, 21.7107) -> (-6.2528, 21.4301)
  line L664 (-6.2528, 21.4301) -> (-7.4212, 21.0402)
  line L665 (-7.4212, 21.0402) -> (-7.2044, 20.3906)
  line L666 (-7.2044, 20.3906) -> (-6.1148, 20.7543)
  line L667 (-6.1148, 20.7543) -> (-6.0212, 20.4737)
  line L668 (-6.0212, 20.4737) -> (-7.1108, 20.11)
  line L669 (-7.1108, 20.11) -> (-6.8171, 19.2299)
  line L670 (-6.8171, 19.2299) -> (-5.6487, 19.6198)
  line L671 (-5.6487, 19.6198) -> (-5.555, 19.3392)
  line L672 (-5.555, 19.3392) -> (-7.0386, 18.8441)
  line L673 (-5.4663, 19.3749) -> (-5.1949, 21.9992)
  line L674 (-5.1949, 21.9992) -> (-4.7957, 22.0894)
  line L675 (-4.7957, 22.0894) -> (-3.4229, 19.8364)
  line L676 (-3.4229, 19.8364) -> (-3.7648, 19.7592)
  line L677 (-3.7648, 19.7592) -> (-4.1401, 20.391)
  line L678 (-4.1401, 20.391) -> (-5.0709, 20.1808)
  line L679 (-5.0709, 20.1808) -> (-5.1382, 19.449)
  line L680 (-5.1382, 19.449) -> (-5.4663, 19.3749)
  line L681 (-4.2915, 20.6476) -> (-4.9283, 21.7105)
  line L682 (-4.9283, 21.7105) -> (-5.0444, 20.4775)
  line L683 (-5.0444, 20.4775) -> (-4.2915, 20.6476)
  line L684 (-1.2342, 20.0966) -> (-1.6628, 20.0462)
  line L685 (-1.6628, 20.0462) -> (-2.5637, 20.9418)
  line L686 (-2.5637, 20.9418) -> (-2.942, 20.8973)
  line L687 (-2.942, 20.8973) -> (-2.8258, 19.9094)
  line L688 (-2.8258, 19.9094) -> (-3.1558, 19.8706)
  line L689 (-3.1558, 19.8706) -> (-3.4477, 22.3535)
  line L690 (-3.4477, 22.3535) -> (-2.8079, 22.4287)
  spline S362 degree 2 poles (-2.8079, 22.4287) (-2.5946, 22.4538) (-2.3015, 22.4414) (-2.1607, 22.3722) knots 0 0 0 1 2 2 2
  spline S363 degree 2 poles (-2.1607, 22.3722) (-2.02, 22.3031) (-1.8381, 22.0573) (-1.8152, 21.8621) knots 0 0 0 1 2 2 2
  spline S364 degree 2 poles (-1.8152, 21.8621) (-1.7832, 21.5905) (-2.0176, 21.1896) (-2.2446, 21.0732) knots 0 0 0 1 2 2 2
  line L691 (-2.2446, 21.0732) -> (-1.2342, 20.0966)
  spline S365 degree 2 poles (-2.1562, 21.7955) (-2.1689, 21.9041) (-2.265, 22.0621) (-2.3519, 22.107) knots 0 0 0 1 2 2 2
  spline S366 degree 2 poles (-2.3519, 22.107) (-2.4278, 22.145) (-2.6194, 22.1612) (-2.7562, 22.1451) knots 0 0 0 1 2 2 2
  line L692 (-2.7562, 22.1451) -> (-3.0842, 22.1066)
  line L693 (-3.0842, 22.1066) -> (-2.9744, 21.173)
  line L694 (-2.9744, 21.173) -> (-2.6846, 21.207)
  spline S367 degree 2 poles (-2.6846, 21.207) (-2.5418, 21.2238) (-2.3203, 21.3009) (-2.2511, 21.3886) knots 0 0 0 1 2 2 2
  spline S368 degree 2 poles (-2.2511, 21.3886) (-2.1867, 21.4655) (-2.141, 21.6667) (-2.1562, 21.7955) knots 0 0 0 1 2 2 2
  line L695 (-0.1636, 20.1083) -> (-1.1315, 20.0772)
  line L696 (-1.1315, 20.0772) -> (-1.1397, 20.3323)
  line L697 (-1.1397, 20.3323) -> (-0.8218, 20.3425)
  line L698 (-0.8218, 20.3425) -> (-0.8858, 22.331)
  line L699 (-0.8858, 22.331) -> (-1.2037, 22.3207)
  line L700 (-1.2037, 22.3207) -> (-1.2119, 22.5759)
  line L701 (-1.2119, 22.5759) -> (-0.244, 22.607)
  line L702 (-0.244, 22.607) -> (-0.2358, 22.3519)
  line L703 (-0.2358, 22.3519) -> (-0.5537, 22.3416)
  line L704 (-0.5537, 22.3416) -> (-0.4897, 20.3532)
  line L705 (-0.4897, 20.3532) -> (-0.1718, 20.3634)
  line L706 (-0.1718, 20.3634) -> (-0.1636, 20.1083)
  line L707 (2.0332, 20.0201) -> (1.661, 20.0412)
  line L708 (1.661, 20.0412) -> (0.6789, 22.2561)
  line L709 (0.6789, 22.2561) -> (0.5566, 20.104)
  line L710 (0.5566, 20.104) -> (0.2472, 20.1215)
  line L711 (0.2472, 20.1215) -> (0.389, 22.6175)
  line L712 (0.389, 22.6175) -> (0.8602, 22.5907)
  line L713 (0.8602, 22.5907) -> (1.7532, 20.5575)
  line L714 (1.7532, 20.5575) -> (1.8655, 22.5336)
  line L715 (1.8655, 22.5336) -> (2.175, 22.5161)
  line L716 (2.175, 22.5161) -> (2.0332, 20.0201)
  spline S369 degree 2 poles (3.5595, 19.7367) (3.2979, 19.7818) (2.8923, 20.0163) (2.7644, 20.2048) knots 0 0 0 1 2 2 2
  spline S370 degree 2 poles (2.7644, 20.2048) (2.6369, 20.3954) (2.5546, 20.9071) (2.6086, 21.2206) knots 0 0 0 1 2 2 2
  spline S371 degree 2 poles (2.6086, 21.2206) (2.6599, 21.5181) (2.9089, 21.9603) (3.0936, 22.1011) knots 0 0 0 1 2 2 2
  spline S372 degree 2 poles (3.0936, 22.1011) (3.2712, 22.237) (3.7407, 22.3369) (4.0022, 22.2918) knots 0 0 0 1 2 2 2
  spline S373 degree 2 poles (4.0022, 22.2918) (4.128, 22.2701) (4.3494, 22.195) (4.4477, 22.1451) knots 0 0 0 1 2 2 2
  spline S374 degree 2 poles (4.4477, 22.1451) (4.5274, 22.1067) (4.7159, 21.9837) (4.7723, 21.9411) knots 0 0 0 1 2 2 2
  line L717 (4.7723, 21.9411) -> (4.7041, 21.5458)
  line L718 (4.7041, 21.5458) -> (4.6762, 21.5506)
  spline S375 degree 2 poles (4.6762, 21.5506) (4.6236, 21.6152) (4.5107, 21.7354) (4.4005, 21.812) knots 0 0 0 1 2 2 2
  spline S376 degree 2 poles (4.4005, 21.812) (4.3093, 21.8791) (4.0632, 21.9894) (3.9154, 22.0149) knots 0 0 0 1 2 2 2
  spline S377 degree 2 poles (3.9154, 22.0149) (3.56, 22.0762) (3.0285, 21.6169) (2.9518, 21.1717) knots 0 0 0 1 2 2 2
  spline S378 degree 2 poles (2.9518, 21.1717) (2.9091, 20.9241) (2.9608, 20.5328) (3.0486, 20.3861) knots 0 0 0 1 2 2 2
  spline S379 degree 2 poles (3.0486, 20.3861) (3.1323, 20.2401) (3.4087, 20.0547) (3.5964, 20.0223) knots 0 0 0 1 2 2 2
  spline S380 degree 2 poles (3.5964, 20.0223) (3.7342, 19.9985) (4.0165, 19.9909) (4.1173, 20.0147) knots 0 0 0 1 2 2 2
  line L719 (4.1173, 20.0147) -> (4.2271, 20.6515)
  line L720 (4.2271, 20.6515) -> (3.6561, 20.75)
  line L721 (3.6561, 20.75) -> (3.7057, 21.0375)
  line L722 (3.7057, 21.0375) -> (4.6001, 20.8832)
  line L723 (4.6001, 20.8832) -> (4.4145, 19.8072)
  spline S381 degree 2 poles (4.4145, 19.8072) (4.3478, 19.7899) (4.1214, 19.7405) (4.0271, 19.7301) knots 0 0 0 1 2 2 2
  spline S382 degree 2 poles (4.0271, 19.7301) (3.8991, 19.7152) (3.6972, 19.713) (3.5595, 19.7367) knots 0 0 0 1 2 2 2
  line L724 (6.9164, 19.8819) -> (6.0161, 20.1725)
  line L725 (6.0161, 20.1725) -> (6.1094, 20.4617)
  line L726 (6.1094, 20.4617) -> (7.0098, 20.1711)
  line L727 (7.0098, 20.1711) -> (6.9164, 19.8819)
  line L728 (8.1362, 19.4147) -> (7.2556, 19.7606)
  line L729 (7.2556, 19.7606) -> (7.3667, 20.0434)
  line L730 (7.3667, 20.0434) -> (8.2473, 19.6975)
  line L731 (8.2473, 19.6975) -> (8.1362, 19.4147)
  line L732 (9.3246, 18.8727) -> (8.4671, 19.2726)
  line L733 (8.4671, 19.2726) -> (8.5956, 19.548)
  line L734 (8.5956, 19.548) -> (9.453, 19.1481)
  line L735 (9.453, 19.1481) -> (9.3246, 18.8727)
  spline S383 degree 2 poles (10.7743, 16.9049) (10.6171, 17.005) (10.419, 17.2634) (10.384, 17.4083) knots 0 0 0 1 2 2 2
  spline S384 degree 2 poles (10.384, 17.4083) (10.3496, 17.5503) (10.4055, 17.8414) (10.4893, 17.973) knots 0 0 0 1 2 2 2
  spline S385 degree 2 poles (10.4893, 17.973) (10.5982, 18.1438) (10.9639, 18.3143) (11.1926, 18.2887) knots 0 0 0 1 2 2 2
  line L736 (11.1926, 18.2887) -> (11.1981, 18.2972)
  spline S386 degree 2 poles (11.1981, 18.2972) (11.1003, 18.4869) (11.0872, 18.798) (11.1895, 18.9586) knots 0 0 0 1 2 2 2
  spline S387 degree 2 poles (11.1895, 18.9586) (11.3409, 19.196) (11.9022, 19.2851) (12.1789, 19.1087) knots 0 0 0 1 2 2 2
  spline S388 degree 2 poles (12.1789, 19.1087) (12.466, 18.9258) (12.6211, 18.4041) (12.4709, 18.1683) knots 0 0 0 1 2 2 2
  spline S389 degree 2 poles (12.4709, 18.1683) (12.3805, 18.0265) (12.0384, 17.8554) (11.8328, 17.8759) knots 0 0 0 1 2 2 2
  line L737 (11.8328, 17.8759) -> (11.8274, 17.8673)
  spline S390 degree 2 poles (11.8274, 17.8673) (11.9574, 17.6643) (11.9903, 17.2974) (11.8662, 17.1027) knots 0 0 0 1 2 2 2
  spline S391 degree 2 poles (11.8662, 17.1027) (11.6941, 16.8327) (11.0682, 16.7176) (10.7743, 16.9049) knots 0 0 0 1 2 2 2
  spline S392 degree 2 poles (11.5583, 17.2604) (11.6411, 17.3903) (11.6365, 17.6094) (11.5414, 17.7805) knots 0 0 0 1 2 2 2
  spline S393 degree 2 poles (11.5414, 17.7805) (11.511, 17.8383) (11.3907, 18.0039) (11.316, 18.1092) knots 0 0 0 1 2 2 2
  spline S394 degree 2 poles (11.316, 18.1092) (11.1509, 18.1063) (10.8802, 17.9569) (10.7877, 17.8117) knots 0 0 0 1 2 2 2
  spline S395 degree 2 poles (10.7877, 17.8117) (10.6657, 17.6203) (10.7374, 17.2239) (10.9116, 17.1128) knots 0 0 0 1 2 2 2
  spline S396 degree 2 poles (10.9116, 17.1128) (11.0893, 16.9996) (11.4407, 17.0759) (11.5583, 17.2604) knots 0 0 0 1 2 2 2
  spline S397 degree 2 poles (12.1919, 18.3413) (12.2823, 18.4831) (12.2135, 18.7936) (12.0444, 18.9014) knots 0 0 0 1 2 2 2
  spline S398 degree 2 poles (12.0444, 18.9014) (11.8906, 18.9994) (11.5864, 18.9555) (11.4938, 18.8103) knots 0 0 0 1 2 2 2
  spline S399 degree 2 poles (11.4938, 18.8103) (11.4274, 18.7061) (11.4356, 18.4966) (11.4994, 18.3743) knots 0 0 0 1 2 2 2
  spline S400 degree 2 poles (11.4994, 18.3743) (11.5269, 18.3231) (11.6546, 18.124) (11.7128, 18.0532) knots 0 0 0 1 2 2 2
  spline S401 degree 2 poles (11.7128, 18.0532) (11.8957, 18.0688) (12.1103, 18.2132) (12.1919, 18.3413) knots 0 0 0 1 2 2 2
  spline S402 degree 2 poles (13.4848, 16.0068) (13.3667, 15.8548) (13.0657, 15.6756) (12.9138, 15.6551) knots 0 0 0 1 2 2 2
  spline S403 degree 2 poles (12.9138, 15.6551) (12.755, 15.6323) (12.4609, 15.7095) (12.3281, 15.8127) knots 0 0 0 1 2 2 2
  spline S404 degree 2 poles (12.3281, 15.8127) (12.1953, 15.9159) (12.0458, 16.1758) (12.0322, 16.33) knots 0 0 0 1 2 2 2
  spline S405 degree 2 poles (12.0322, 16.33) (12.0132, 16.5167) (12.1777, 16.9662) (12.3816, 17.2285) knots 0 0 0 1 2 2 2
  spline S406 degree 2 poles (12.3816, 17.2285) (12.5818, 17.4861) (13.0093, 17.8183) (13.2391, 17.8861) knots 0 0 0 1 2 2 2
  spline S407 degree 2 poles (13.2391, 17.8861) (13.4631, 17.9532) (13.9327, 17.8576) (14.1551, 17.6847) knots 0 0 0 1 2 2 2
  spline S408 degree 2 poles (14.1551, 17.6847) (14.2207, 17.6338) (14.3259, 17.5315) (14.3579, 17.4835) knots 0 0 0 1 2 2 2
  line L738 (14.3579, 17.4835) -> (14.1602, 17.2292)
  line L739 (14.1602, 17.2292) -> (14.149, 17.2379)
  spline S409 degree 2 poles (14.149, 17.2379) (14.1272, 17.2856) (14.0189, 17.4237) (13.9421, 17.4833) knots 0 0 0 1 2 2 2
  spline S410 degree 2 poles (13.9421, 17.4833) (13.6958, 17.6748) (13.1349, 17.5771) (12.8524, 17.2731) knots 0 0 0 1 2 2 2
  spline S411 degree 2 poles (12.8524, 17.2731) (12.9978, 17.2653) (13.2521, 17.1832) (13.3705, 17.0912) knots 0 0 0 1 2 2 2
  spline S412 degree 2 poles (13.3705, 17.0912) (13.4856, 17.0017) (13.6223, 16.821) (13.662, 16.6773) knots 0 0 0 1 2 2 2
  spline S413 degree 2 poles (13.662, 16.6773) (13.7074, 16.5111) (13.6165, 16.1763) (13.4848, 16.0068) knots 0 0 0 1 2 2 2
  spline S414 degree 2 poles (13.2073, 16.2045) (13.3018, 16.326) (13.3659, 16.5405) (13.3402, 16.6528) knots 0 0 0 1 2 2 2
  spline S415 degree 2 poles (13.3402, 16.6528) (13.3198, 16.7354) (13.2097, 16.8646) (13.141, 16.918) knots 0 0 0 1 2 2 2
  spline S416 degree 2 poles (13.141, 16.918) (13.0482, 16.9901) (12.8303, 17.0696) (12.7045, 17.0828) knots 0 0 0 1 2 2 2
  spline S417 degree 2 poles (12.7045, 17.0828) (12.6805, 17.0552) (12.6351, 17.0033) (12.6027, 16.9617) knots 0 0 0 1 2 2 2
  spline S418 degree 2 poles (12.6027, 16.9617) (12.4436, 16.757) (12.3284, 16.4437) (12.3382, 16.3308) knots 0 0 0 1 2 2 2
  spline S419 degree 2 poles (12.3382, 16.3308) (12.3457, 16.2249) (12.4287, 16.0809) (12.4975, 16.0274) knots 0 0 0 1 2 2 2
  spline S420 degree 2 poles (12.4975, 16.0274) (12.6575, 15.9031) (13.0308, 15.9773) (13.2073, 16.2045) knots 0 0 0 1 2 2 2
  line L740 (14.6071, 15.7787) -> (14.3102, 16.0485)
  line L741 (14.3102, 16.0485) -> (14.6317, 16.4023)
  line L742 (14.6317, 16.4023) -> (14.9286, 16.1326)
  line L743 (14.9286, 16.1326) -> (14.6071, 15.7787)
  line L744 (13.6671, 14.7441) -> (13.3702, 15.0138)
  line L745 (13.3702, 15.0138) -> (13.6917, 15.3677)
  line L746 (13.6917, 15.3677) -> (13.9886, 15.098)
  line L747 (13.9886, 15.098) -> (13.6671, 14.7441)
  line L748 (15.0743, 13.3168) -> (14.2373, 14.2038)
  line L749 (14.2373, 14.2038) -> (14.423, 14.379)
  line L750 (14.423, 14.379) -> (14.7344, 14.049)
  line L751 (14.7344, 14.049) -> (15.953, 15.1989)
  line L752 (15.953, 15.1989) -> (15.6415, 15.5289)
  line L753 (15.6415, 15.5289) -> (15.808, 15.6861)
  spline S421 degree 2 poles (15.808, 15.6861) (15.9846, 15.4989) (16.2575, 15.4222) (16.416, 15.5495) knots 0 0 0 1 2 2 2
  line L754 (16.416, 15.5495) -> (16.594, 15.3609)
  line L755 (16.594, 15.3609) -> (14.9555, 13.8147)
  line L756 (14.9555, 13.8147) -> (15.26, 13.492)
  line L757 (15.26, 13.492) -> (15.0743, 13.3168)
  constraints: 1 centre point, 1 coincident, 1 other